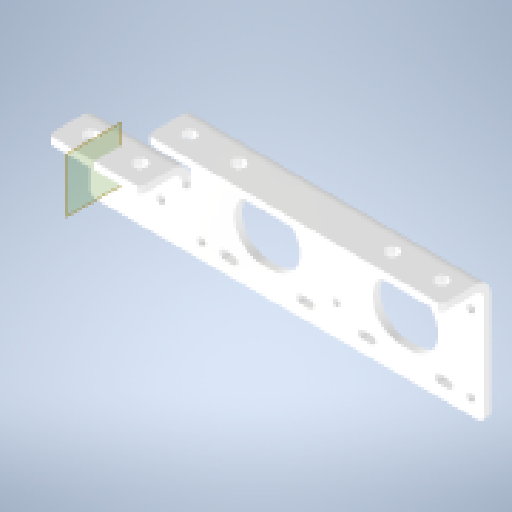
# Autodesk Inventor part: XY Motor Mount A
Saved by Autodesk Inventor 2024 (Build 280153000, 153)
## iProperties
Created: 2024-12-26
Part Number: XY Motor Mount A
Material: Aluminum 6061
Document SubType Name: Sheet Metal
Designer: Ishaan
Density: 2.7 g/cm^3
Sheet Metal Rule: Default
Appearance: Aluminum - Flat
Author: Ishaan
Autodesk Inventor part; units mm, degrees
sketch "Sketch1" plane through (0, 0, 0) normal (0, 0, 1) x (1, 0, 0)
  line L0 (20, -10) -> (-20, -10) construction
  line L1 (-20, -10) -> (-20, 10) construction
  line L2 (-20, 10) -> (20, 10) construction
  line L3 (20, 10) -> (20, -10) construction
  line L4 (20, -10) -> (-20, 10) construction
  line L5 (-20, -10) -> (20, 10) construction
  line L6 (-18.5, -10) -> (18.5, -10)
  line L7 (18.5, -10) -> (18.5, -40)
  line L8 (18.5, -40) -> (-18.5, -40)
  line L9 (-18.5, -40) -> (-18.5, -10)
  line L10 (21.5, 10) -> (140.5, 10)
  line L11 (140.5, 10) -> (140.5, -40)
  line L12 (140.5, -40) -> (21.5, -40)
  line L13 (21.5, -40) -> (21.5, 10)
  line L14 (18.5, -18) -> (21.5, -18)
  line L15 (21.5, -18) -> (21.5, -40)
  line L16 (21.5, -40) -> (18.5, -40)
  line L17 (18.5, -40) -> (18.5, -18)
  circle A0 centre (-8.764, -25) radius 6.365 construction
  circle A1 centre (-8.764, -25) radius 6.736 construction
  circle A2 centre (10.236, -27) radius 6 construction
  line L18 (74.5, -39.5) -> (31.5, -39.5) construction
  line L19 (31.5, -39.5) -> (31.5, 3.5) construction
  line L20 (31.5, 3.5) -> (74.5, 3.5) construction
  line L21 (74.5, 3.5) -> (74.5, -39.5) construction
  line L22 (74.5, -39.5) -> (31.5, 3.5) construction
  line L23 (31.5, -39.5) -> (74.5, 3.5) construction
  line L24 (130.5, -39.5) -> (87.5, -39.5) construction
  line L25 (87.5, -39.5) -> (87.5, 3.5) construction
  line L26 (87.5, 3.5) -> (130.5, 3.5) construction
  line L27 (130.5, 3.5) -> (130.5, -39.5) construction
  line L28 (130.5, -39.5) -> (87.5, 3.5) construction
  line L29 (87.5, -39.5) -> (130.5, 3.5) construction
  line L30 (74.5, -18) -> (87.5, -18) construction
  line L31 (26.5, -18) -> (135.5, -18) construction
  line L32 (68.5, -33.5) -> (37.5, -33.5) construction
  line L33 (37.5, -33.5) -> (37.5, -2.5) construction
  line L34 (37.5, -2.5) -> (68.5, -2.5) construction
  line L35 (68.5, -2.5) -> (68.5, -33.5) construction
  line L36 (68.5, -33.5) -> (37.5, -2.5) construction
  line L37 (37.5, -33.5) -> (68.5, -2.5) construction
  line L38 (135.5, -2.5) -> (135.5, -33.5) construction
  line L39 (26.5, -2.5) -> (26.5, -33.5) construction
  line L40 (81, -8.5) -> (81, -27.5) construction
  line L41 (124.5, -33.5) -> (93.5, -33.5) construction
  line L42 (93.5, -33.5) -> (93.5, -2.5) construction
  line L43 (93.5, -2.5) -> (124.5, -2.5) construction
  line L44 (124.5, -2.5) -> (124.5, -33.5) construction
  line L45 (124.5, -33.5) -> (93.5, -2.5) construction
  line L46 (93.5, -33.5) -> (124.5, -2.5) construction
  circle A3 centre (-8.764, -25) radius 9.736 construction
  circle A4 centre (10.236, -27) radius 9.736 construction
  point P0 (0, 0)
  point P1 (0, -10)
  point P2 (20, -18)
  point P3 (53, -18)
  point P4 (109, -18)
  point P5 (68.5, -2.5)
  point P6 (81, -18)
  point P7 (21.5, -18)
  point P8 (-18.5, -32.7888)
  point P9 (-18.5, -25)
  dimension "d0" = 40
  dimension "d1" = 20
  dimension "d2" = 37
  dimension "d3" = 50
  dimension "d4" = 8
  dimension "d7" = 15
  dimension "d8" = 12.73
  dimension "d9" = 0.371
  dimension "d10" = 3
  dimension "d11" = 12
  dimension "d12" = 2
  dimension "d13" = 19
  dimension "d14" = 43
  dimension "d15" = 43
  dimension "d16" = 28
  dimension "d18" = 56
  dimension "d19" = 13
  dimension "d20" = 10
  dimension "d21" = 10
  dimension "d22" = 5
  dimension "d23" = 31
  dimension "d24" = 31
  dimension "d80" = 19
  constraints: 94 end point, 20 midpoint, 17 coincident, 16 parallel, 9 horizontal, 8 perpendicular, 6 equal length, 5 centre point, 3 point on line, 3 vertical, 2 collinear, 1 equal radius, 1 horizontal alignment, 1 tangent, 1 vertical alignment
  measures "d0" distance of L1.end L2.end
  measures "d1" distance of L0.end L1.end
  measures "d2" distance between parallel lines of L7 L9
  measures "d3" distance between parallel lines of L8 L2
  measures "d4" distance between parallel lines of L0 L14
  measures "d7" distance from line of point (-8.764, -25) L6
  measures "d8" diameter of A0
  measures "d9" radial gap between concentric circles of A0 A1
  measures "d10" distance edge to line of A1 L9
  measures "d11" diameter of A2
  measures "d12" vertical distance of A0.centre A2.centre
  measures "d13" horizontal distance of A2.centre A0.centre
  measures "d14" distance of L19.end L20.end
  measures "d15" distance of L18.end L19.end
  measures "d16" distance from line of point (53, -18) L2
  measures "d18" distance of point (109, -18) point (53, -18)
  measures "d19" distance between parallel lines of L25 L21
  measures "d20" distance between parallel lines of L11 L27
  measures "d21" distance between parallel lines of L19 L13
  measures "d22" distance from line of L31.start L19
  measures "d23" distance of L33.end L34.end
  measures "d24" distance of L32.end L33.end
  measures "d80" distance of L40.start L40.end
extrude "Plate1" add sketch "Sketch1" along normal blind 3.048
sketch "Sketch2" plane through (-18.5, -13.048, 0) normal (0, 1, 0) x (-1, 0, 0)
  line L0 (-37, 0) -> (0, 0)
  line L1 (0, 0) -> (0, 20.048)
  line L2 (0, 20.048) -> (-37, 20.048)
  line L3 (-37, 20.048) -> (-37, 0)
  constraints: 6 end point, 1 horizontal, 1 perpendicular, 1 vertical
edge flange "Flange1" height 17 angle 90 thickness 3.048 bend radius 3.048 thickness toward (0, 1, 0) relief tear relief width 3.048 relief depth 1.524 edges at (0, -10, 3.048) wall of the first edge with corners at (18.5, -13.048, 0) (-18.5, -13.048, 0) (-18.5, -13.048, 20.048) (18.5, -13.048, 20.048)
bend "Bend1"
corner "Corner1"
sketch "Sketch3" plane through (21.5, 6.952, 0) normal (0, 1, 0) x (-1, 0, 0)
  line L0 (-119, 0) -> (0, 0)
  line L1 (0, 0) -> (0, 20.048)
  line L2 (0, 20.048) -> (-119, 20.048)
  line L3 (-119, 20.048) -> (-119, 0)
  constraints: 6 end point, 1 horizontal, 1 perpendicular, 1 vertical
edge flange "Flange2" height 17 angle 90 thickness 3.048 bend radius 3.048 thickness toward (0, 1, 0) relief tear relief width 3.048 relief depth 1.524 edges at (81, 10, 3.048) wall of the first edge with corners at (140.5, 6.952, 0) (21.5, 6.952, 0) (21.5, 6.952, 20.048) (140.5, 6.952, 20.048)
bend "Bend2"
corner "Corner2"
hole "Hole1" at (-8.764, -25, 0) at (10.236, -27, 0) at (37.5, -2.5, 0) at (68.5, -2.5, 0) at (68.5, -33.5, 0) at (37.5, -33.5, 0) at (81, -8.5, 0) at (26.5, -2.5, 0) at (26.5, -33.5, 0) at (81, -27.5, 0) at (135.5, -2.5, 0) at (135.5, -33.5, 0) at (93.5, -2.5, 0) at (124.5, -2.5, 0) at (124.5, -33.5, 0) at (93.5, -33.5, 0) direction (0, 0, 1) diameter 3.3 end through all
fillet "Fillet1" radius 1 2 edges at (18.5, -18, 1.524) (21.5, -18, 1.524)
sketch "Sketch4" plane through (-18.5, -13.048, 20.048) normal (0, -1, 0) x (1, 0, 0)
  line L0 (37, 0) -> (0, 0) construction
  line L1 (28.5, 0) -> (28.5, -8.5) construction
  line L2 (0, 0) -> (8.5, 0) construction
  line L3 (8.5, 0) -> (8.5, -8.5) construction
  line L4 (8.5, -8.5) -> (0, -8.5) construction
  line L5 (0, -8.5) -> (0, 0) construction
  line L6 (8.5, -8.5) -> (28.5, -8.5) construction
  point P0 (18.5, -20.048)
  point P1 (18.5, 0)
  point P2 (18.5, -8.5)
  dimension "d56" = 20
  constraints: 12 end point, 2 coincident, 2 horizontal, 2 midpoint, 2 parallel, 2 perpendicular, 1 vertical alignment
  measures "d56" distance between parallel lines of L1 L3
hole "Hole2" at (-10, -13.048, 11.548) at (10, -13.048, 11.548) direction (0, 1, 0) diameter 5.4 end through all
sketch "Sketch5" plane through (21.5, 6.952, 20.048) normal (0, -1, 0) x (1, 0, 0)
  line L0 (0, -13.952) -> (119, -13.952) projected
  line L1 (119, -13.952) -> (119, 0) projected
  line L2 (119, 0) -> (0, 0) projected
  line L3 (0, -13.952) -> (0, 0) projected
  circle A0 centre (-11.5, -8.5) radius 2.7 projected
  line L4 (110.5, -8.5) -> (119, -8.5) construction
  line L5 (119, -8.5) -> (119, 0) construction
  line L6 (119, 0) -> (110.5, 0) construction
  line L7 (110.5, 0) -> (110.5, -8.5) construction
  line L8 (8.5, -8.5) -> (0, -8.5) construction
  line L9 (0, -8.5) -> (0, 0) construction
  line L10 (0, 0) -> (8.5, 0) construction
  line L11 (8.5, 0) -> (8.5, -8.5) construction
  point P0 (-21.5, -20.048)
  point P1 (28.5, -8.5)
  point P2 (90.5, -8.5)
  dimension "d64" = 20
  dimension "d65" = 20
  constraints: 16 end point, 4 horizontal alignment, 4 parallel, 4 perpendicular, 2 horizontal
  measures "d64" distance of L4.start point (90.5, -8.5)
  measures "d65" distance of point (28.5, -8.5) L8.start
hole "Hole3" at (30, 6.952, 11.548) at (50, 6.952, 11.548) at (132, 6.952, 11.548) at (112, 6.952, 11.548) direction (0, 1, 0) diameter 5.4 end through all
fillet "Fillet2" radius 2 6 edges at (140.5, 8.476, 20.048) (-18.5, -11.524, 20.048) (18.5, -11.524, 20.048) (21.5, 8.476, 20.048) (140.5, -40, 1.524) (-18.5, -40, 1.524)
sketch "Sketch6" plane through (0, 0, 3.048) normal (0, 0, 1) x (1, 0, 0)
  line L0 (138.5, -40) -> (-16.5, -40) construction
  arc A0 (138.5, -40) -> (140.5, -38) centre (138.5, -38) ccw construction
  line L1 (140.5, 3.904) -> (140.5, -38) construction
  line L2 (140.5, 3.904) -> (21.5, 3.904) construction
  line L3 (21.5, -17) -> (21.5, 3.904) construction
  arc A1 (20.5, -18) -> (21.5, -17) centre (20.5, -17) ccw construction
  line L4 (19.5, -18) -> (20.5, -18) construction
  arc A2 (18.5, -17) -> (19.5, -18) centre (19.5, -17) ccw construction
  circle A3 centre (93.5, -33.5) radius 1.65 construction
  circle A4 centre (124.5, -33.5) radius 1.65 construction
  circle A5 centre (124.5, -2.5) radius 1.65 construction
  circle A6 centre (93.5, -2.5) radius 1.65 construction
  circle A7 centre (135.5, -33.5) radius 1.65 construction
  circle A8 centre (135.5, -2.5) radius 1.65 construction
  circle A9 centre (81, -27.5) radius 1.65 construction
  circle A10 centre (26.5, -33.5) radius 1.65 construction
  circle A11 centre (26.5, -2.5) radius 1.65 construction
  circle A12 centre (81, -8.5) radius 1.65 construction
  circle A13 centre (37.5, -33.5) radius 1.65 construction
  circle A14 centre (68.5, -33.5) radius 1.65 construction
  circle A15 centre (68.5, -2.5) radius 1.65 construction
  circle A16 centre (37.5, -2.5) radius 1.65 construction
  line L5 (68.5, -33.5) -> (37.5, -33.5) construction
  line L6 (37.5, -33.5) -> (37.5, -2.5) construction
  line L7 (37.5, -2.5) -> (68.5, -2.5) construction
  line L8 (68.5, -2.5) -> (68.5, -33.5) construction
  line L9 (68.5, -33.5) -> (37.5, -2.5) construction
  line L10 (37.5, -33.5) -> (68.5, -2.5) construction
  line L11 (124.5, -33.5) -> (93.5, -33.5) construction
  line L12 (93.5, -33.5) -> (93.5, -2.5) construction
  line L13 (93.5, -2.5) -> (124.5, -2.5) construction
  line L14 (124.5, -2.5) -> (124.5, -33.5) construction
  line L15 (124.5, -33.5) -> (93.5, -2.5) construction
  line L16 (93.5, -33.5) -> (124.5, -2.5) construction
  line L17 (35.5, -2.5) -> (39.5, -2.5) construction
  line L18 (35.5, -4.15) -> (39.5, -4.15)
  line L19 (39.5, -0.85) -> (35.5, -0.85)
  arc A17 (35.5, -0.85) -> (35.5, -4.15) centre (35.5, -2.5) ccw
  arc A18 (39.5, -4.15) -> (39.5, -0.85) centre (39.5, -2.5) ccw
  line L20 (51, -18) -> (55, -18) construction
  line L21 (51, -29.25) -> (55, -29.25)
  line L22 (55, -6.75) -> (51, -6.75)
  arc A19 (51, -6.75) -> (51, -29.25) centre (51, -18) ccw
  arc A20 (55, -29.25) -> (55, -6.75) centre (55, -18) ccw
  line L23 (107, -18) -> (111, -18) construction
  line L24 (107, -29.25) -> (111, -29.25)
  line L25 (111, -6.75) -> (107, -6.75)
  arc A21 (107, -6.75) -> (107, -29.25) centre (107, -18) ccw
  arc A22 (111, -29.25) -> (111, -6.75) centre (111, -18) ccw
  line L26 (18.5, -16.096) -> (18.5, -17) projected
  line L27 (18.5, -16.096) -> (-18.5, -16.096) projected
  line L28 (-18.5, -38) -> (-18.5, -16.096) projected
  arc A23 (-18.5, -38) -> (-16.5, -40) centre (-16.5, -38) ccw projected
  point P0 (0, 0)
  point P1 (53, -18)
  point P2 (109, -18)
  dimension "d74" = 4
  dimension "d77" = 22.5
  constraints: 48 end point, 13 tangent, 12 point on circle, 7 midpoint, 7 parallel, 6 centre point, 5 coincident, 4 horizontal, 2 equal length, 2 perpendicular, 1 equal radius, 1 point on line
  measures "d74" distance of L19.start L19.end
  measures "d77" diameter of A20
extrude "Extrusion2" cut sketch "Sketch6" against normal through all contours A17 L19 A18 L18
ref_plane "Work Plane1" through (53, -18, 3.048) normal (1, 0, 0) x (0, 1, 0)
mirror "Mirror1" about plane through (53, -18, 3.048) normal (1, 0, 0) of "Extrusion2"
ref_plane "Work Plane2" through (109, -18, 3.048) normal (1, 0, 0) x (0, 1, 0)
ref_plane "Work Plane3" through (81, -18, 3.048) normal (1, 0, 0) x (0, 1, 0)
mirror "Mirror2" about plane through (81, -18, 3.048) normal (1, 0, 0) of "Extrusion2", "Mirror1"
ref_plane "Work Plane4" through (53, -18, 3.048) normal (0, 1, 0) x (-1, 0, 0)
mirror "Mirror3" about plane through (53, -18, 3.048) normal (0, 1, 0) of "Extrusion2", "Mirror1", "Mirror2"
extrude "Extrusion3" cut sketch "Sketch6" against normal through all contours A19 L22 A20 L21 | A21 L25 A22 L24
ref_plane "Work Plane5" through (0, -13.048, 20.048) normal (-1, 0, 0) x (0, -1, 0)
equation "\"d21\" = d20"
equation "\"d22\" = 0.5 * d21"
equation "\"d51\" = Thickness"
equation "\"d25\" = Thickness"
equation "\"d26\" = BendReliefWidth"
equation "\"d27\" = BendReliefDepth"
equation "\"d28\" = MinimumRemnant"
equation "\"d29\" = TransitionRadius"
equation "\"d32\" = BendRadius"
equation "\"d33\" = CornerReliefSize"
equation "\"d34\" = GapSize"
equation "\"d35\" = JacobiRadiusSize"
equation "\"d36\" = BendReliefWidth"
equation "\"d37\" = BendReliefDepth"
equation "\"d38\" = MinimumRemnant"
equation "\"d39\" = TransitionRadius"
equation "\"d42\" = BendRadius"
equation "\"d43\" = CornerReliefSize"
equation "\"d44\" = GapSize"
equation "\"d45\" = JacobiRadiusSize"
equation "\"BendRadius\" = Thickness"
equation "\"BendReliefWidth\" = Thickness"
equation "\"BendReliefDepth\" = 0.5 * Thickness"
equation "\"CornerReliefSize\" = 4 * Thickness"
equation "\"MinimumRemnant\" = 2 * Thickness"
equation "\"TransitionRadius\" = BendRadius"
equation "\"JacobiRadiusSize\" = BendRadius"
equation "\"GapSize\" = Thickness"
equation "\"Thickness\" = 3.048"
body "Solid1"
